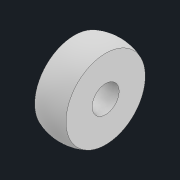
# Autodesk Inventor part: tpu_caster
Saved by Autodesk Inventor 2022 (Build 260153000, 153)
## iProperties
Created: 2023-12-10
Part Number: tpu_caster
Material: 一般
Document SubType Name: Modeling
Designer: gisen
Density: 1 g/cm^3
Appearance: 既定
Author: gisen
Autodesk Inventor part; units mm, degrees
ref_plane "YZ Plane" through (0, 0, 0) normal (1, 0, 0) x (0, 1, 0)
ref_plane "XZ Plane" through (0, 0, 0) normal (0, 1, 0) x (-1, 0, 0)
ref_plane "XY Plane" through (0, 0, 0) normal (0, 0, 1) x (1, 0, 0)
sketch "スケッチ1" plane through (0, 0, 0) normal (0, 0, 1) x (1, 0, 0)
  line L0 (0, 0) -> (20, 0) construction
  line L1 (1.2, 8.6) -> (0, 8.6)
  line L2 (0, 8.6) -> (0, 24) construction
  line L3 (1.2, 8.6) -> (1.2, 7.6)
  line L4 (1.2, 7.6) -> (18.8, 7.6)
  line L5 (18.8, 7.6) -> (18.8, 8.6)
  line L6 (18.8, 8.6) -> (20, 8.6)
  line L7 (20, 8.6) -> (20, 24) construction
  line L8 (20, 24) -> (0, 24) construction
  circle A0 centre (10, 0) radius 24 construction
  arc A1 (20, 21.8174) -> (0, 21.8174) centre (10, 0) ccw
  line L9 (0, 21.8174) -> (0, 8.6)
  line L10 (20, 21.8174) -> (20, 8.6)
  line L11 (18.8, 8.6) -> (18.8, 22.3285)
  line L12 (1.2, 8.6) -> (1.2, 22.3285)
  point P0 (10, 24)
  point P1 (10, 7.6)
  dimension "d0" = 1.2
  dimension "d1" = 20
  dimension "d2" = 1
  dimension "d3" = 7.6
  dimension "d4" = 24
  constraints: 26 end point, 7 point on circle, 6 perpendicular, 3 midpoint, 3 vertical alignment, 2 centre point, 2 collinear, 2 horizontal, 2 point on line, 2 vertical, 1 coincident, 1 horizontal alignment, 1 parallel
  measures "d0" distance of L1.start L1.end
  measures "d1" distance between parallel lines of L7 L2
  measures "d2" distance of L1.start L3.end
  measures "d3" distance between parallel lines of L0 L4
  measures "d4" distance between parallel lines of L0 L8
revolve "回転1" add sketch "スケッチ1" angle 360 about axis through (0, 0, 0) along (1, 0, 0) contours L12 A1 L11 L5 L4 L3
